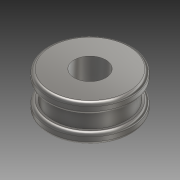
# Autodesk Inventor part: bearing_thrust_3x8x3,5
Saved by Autodesk Inventor 2017 SP1 (Build 210196100, 196)
## iProperties
Created: 2017-08-03
Part Number: bearing_thrust_3x8x3,5
Material: Stainless Steel
Document SubType Name: Modeling
Designer: Tomasz
Density: 8 g/cm^3
Appearance: Semi-Polished
Author: Tomasz
Autodesk Inventor part; units mm, degrees
ref_plane "YZ Plane" through (0, 0, 0) normal (1, 0, 0) x (0, 1, 0)
ref_plane "XZ Plane" through (0, 0, 0) normal (0, 1, 0) x (-1, 0, 0)
ref_plane "XY Plane" through (0, 0, 0) normal (0, 0, 1) x (1, 0, 0)
sketch "Sketch1" plane through (0, 0, 0) normal (1, 0, 0) x (0, 1, 0)
  line L0 (0, 4.1186) -> (0, -3.7432) construction
  line L1 (0, 0) -> (4.3895, 0) construction
  line L2 (1.5, 1.75) -> (1.5, -1.75)
  line L3 (1.5, -1.75) -> (4, -1.75)
  line L4 (4, -1.75) -> (4, -0.75)
  line L5 (4, -0.75) -> (3.5, -0.75)
  line L6 (3.5, -0.75) -> (3.5, 0.75)
  line L7 (3.5, 0.75) -> (4, 0.75)
  line L8 (4, 0.75) -> (4, 1.75)
  line L9 (4, 1.75) -> (1.5, 1.75)
  dimension "d0" = 3.5
  dimension "d1" = 8
  dimension "d2" = 3
  dimension "d3" = 1.5
  dimension "d4" = 0.5
  constraints: 20 end point, 6 perpendicular, 3 point on line, 2 vertical, 1 horizontal, 2 other
  measures "d0" distance between parallel lines of L3 L9
  measures "d1" diameter of L4 L0
  measures "d2" diameter of L2 L0
  measures "d3" distance between parallel lines of L5 L7
  measures "d4" distance between parallel lines of L6 L4
revolve "Revolution1" add sketch "Sketch1" angle 360 about axis through (0, 0, 4.1186) along (0, 0, -1)
fillet "Fillet1" radius 0.3 4 edges at (0, -4, 1.75) (0, -4, -1.75) (0, -4, -0.75) (0, -4, 0.75)
body "Solid1"
